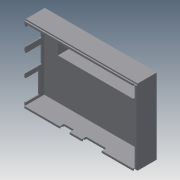
# Autodesk Inventor part: raspi_enclosure2
Saved by Autodesk Inventor 2015 (Build 190159000, 159)
## iProperties
Created: 2018-01-16
Part Number: raspi_enclosure2
Material: Generic
Document SubType Name: Modeling
Designer: rissa
Density: 1 g/cm^3
Appearance: Default
Author: rissa
Autodesk Inventor part; units mm, degrees
ref_plane "YZ Plane" through (0, 0, 0) normal (1, 0, 0) x (0, 1, 0)
ref_plane "XZ Plane" through (0, 0, 0) normal (0, 1, 0) x (-1, 0, 0)
ref_plane "XY Plane" through (0, 0, 0) normal (0, 0, 1) x (1, 0, 0)
sketch "Sketch1" plane through (0, 0, 0) normal (0, 0, 1) x (1, 0, 0)
  line L0 (-43.7903, 41.0199) -> (46.7097, 41.0199)
  line L1 (46.7097, 41.0199) -> (46.7097, -19.9801)
  line L2 (46.7097, -19.9801) -> (-43.7903, -19.9801)
  line L3 (-43.7903, -19.9801) -> (-43.7903, 41.0199)
  point P0 (0, 0)
  dimension "d0" = 90.5
  dimension "d1" = 61
  constraints: 8 end point, 2 parallel, 1 horizontal, 1 perpendicular
  measures "d0" distance of L0.start L0.end
  measures "d1" distance between parallel lines of L2 L0
extrude "Extrusion1" add sketch "Sketch1" along normal blind 1.5
sketch "Sketch2" plane through (0, 0, 1.5) normal (0, 0, 1) x (1, 0, 0)
  line L0 (-42.7903, 39.5199) -> (45.2097, 39.5199)
  line L1 (45.2097, 39.5199) -> (45.2097, -18.4801)
  line L2 (45.2097, -18.4801) -> (-42.7903, -18.4801)
  line L3 (-42.7903, -18.4801) -> (-42.7903, 39.5199)
  line L4 (-43.7903, 41.0199) -> (46.7097, 41.0199)
  line L5 (46.7097, 41.0199) -> (46.7097, -19.9801)
  line L6 (46.7097, -19.9801) -> (-43.7903, -19.9801)
  line L7 (-43.7903, -19.9801) -> (-43.7903, 41.0199)
  point P0 (0, 0)
  dimension "d4" = 1.5
  dimension "d5" = 1.5
  dimension "d6" = 1.5
  dimension "d7" = 1
  constraints: 16 end point, 4 parallel, 2 horizontal, 2 perpendicular
  measures "d4" distance between parallel lines of L4 L0
  measures "d5" distance between parallel lines of L5 L1
  measures "d6" distance between parallel lines of L6 L2
  measures "d7" distance between parallel lines of L3 L7
extrude "Extrusion2" add sketch "Sketch2" along normal blind 16
sketch "Sketch3" plane through (-43.7903, -19.9801, 0) normal (-1, 0, 0) x (0, 0, 1)
  line L0 (17.5, 1.5) -> (17.5, 59.5) projected
  line L1 (17.5, 20.5) -> (5.5, 20.5)
  line L2 (5.5, 20.5) -> (5.5, 3.5)
  line L3 (5.5, 3.5) -> (17.5, 3.5)
  line L4 (17.5, 3.5) -> (17.5, 20.5)
  line L5 (17.5, 38) -> (3.5, 38)
  line L6 (3.5, 38) -> (3.5, 24)
  line L7 (3.5, 24) -> (17.5, 24)
  line L8 (17.5, 24) -> (17.5, 38)
  line L9 (17.5, 56.5) -> (3.5, 56.5)
  line L10 (3.5, 56.5) -> (3.5, 42.5)
  line L11 (3.5, 42.5) -> (17.5, 42.5)
  line L12 (17.5, 42.5) -> (17.5, 56.5)
  line L13 (0, 0) -> (17.5, 0) projected
  point P0 (0, 19.9801)
  dimension "d10" = 3.5
  dimension "d11" = 12
  dimension "d12" = 17
  dimension "d13" = 3.5
  dimension "d14" = 14
  dimension "d15" = 14
  dimension "d16" = 14
  dimension "d17" = 4.5
  dimension "d18" = 14
  constraints: 24 end point, 6 parallel, 3 horizontal, 3 perpendicular, 3 point on line
  measures "d10" distance between parallel lines of L13 L3
  measures "d11" distance between parallel lines of L2 L0
  measures "d12" distance between parallel lines of L3 L1
  measures "d13" distance between parallel lines of L7 L1
  measures "d14" distance between parallel lines of L8 L6
  measures "d15" distance between parallel lines of L7 L5
  measures "d16" distance between parallel lines of L11 L9
  measures "d17" distance between parallel lines of L5 L11
  measures "d18" distance between parallel lines of L0 L10
extrude "Extrusion3" cut sketch "Sketch3" against normal blind 1
sketch "Sketch4" plane through (0, 0, 1.5) normal (0, 0, 1) x (1, 0, 0)
  line L0 (45.2097, 39.5199) -> (-15.7903, 39.5199)
  line L1 (-15.7903, 39.5199) -> (-15.7903, 30.5199)
  line L2 (-15.7903, 30.5199) -> (45.2097, 30.5199)
  line L3 (45.2097, 30.5199) -> (45.2097, 39.5199)
  point P0 (0, 0)
  dimension "d21" = 61
  dimension "d22" = 9
  constraints: 8 end point, 2 parallel, 1 horizontal, 1 perpendicular
  measures "d21" distance between parallel lines of L1 L3
  measures "d22" distance between parallel lines of L0 L2
extrude "Extrusion4" cut sketch "Sketch4" against normal blind 1.5
sketch "Sketch5" plane through (0, 0, 1.5) normal (0, 0, 1) x (1, 0, 0)
  line L0 (45.2097, 30.5199) -> (-15.7903, 30.5199)
  line L1 (-15.7903, 30.5199) -> (-15.7903, 29.0199)
  line L2 (-15.7903, 29.0199) -> (45.2097, 29.0199)
  line L3 (45.2097, 29.0199) -> (45.2097, 30.5199)
  line L4 (-42.7903, 39.5199) -> (45.2097, 39.5199) projected
  line L5 (-15.7903, 29.0199) -> (-17.2903, 29.0199)
  line L6 (-17.2903, 29.0199) -> (-17.2903, 39.5199)
  line L7 (-17.2903, 39.5199) -> (-15.7903, 39.5199)
  line L8 (-15.7903, 39.5199) -> (-15.7903, 29.0199)
  line L9 (46.7097, 41.0199) -> (46.7097, -19.9801) projected
  line L10 (45.2097, -18.4801) -> (45.2097, 30.5199) projected
  point P0 (0, 0)
  dimension "d25" = 1.5
  dimension "d26" = 1.5
  dimension "d28" = 61
  dimension "d29" = 9
  constraints: 16 end point, 4 parallel, 2 horizontal, 2 perpendicular, 1 point on line
  measures "d25" distance between parallel lines of L2 L0
  measures "d26" distance between parallel lines of L8 L6
  measures "d28" distance between parallel lines of L8 L10
  measures "d29" distance between parallel lines of L4 L0
extrude "Extrusion5" add sketch "Sketch5" along normal blind 16
sketch "Sketch6" plane through (0, 0, 17.5) normal (0, 0, 1) x (1, 0, 0)
  line L0 (-43.7903, 0.5199) -> (-42.7903, 0.5199) projected
  line L1 (-42.7903, 4.0199) -> (-43.7903, 4.0199) projected
  line L2 (-42.7903, 0.5199) -> (-42.7903, 4.0199) projected
  line L3 (-43.7903, 4.0199) -> (-43.7903, 0.5199) projected
  line L4 (-43.7903, -19.9801) -> (-43.7903, 41.0199) projected
  line L5 (-43.2903, 4.0199) -> (-43.7903, 4.0199)
  line L6 (-43.7903, 4.0199) -> (-43.7903, 3.0199)
  line L7 (-43.7903, 3.0199) -> (-43.2903, 3.0199)
  line L8 (-43.2903, 3.0199) -> (-43.2903, 4.0199)
  point P0 (0, 0)
  dimension "d32" = 3.5
  dimension "d33" = 1
  dimension "d34" = 0.5
  dimension "d35" = 1
  constraints: 8 end point, 2 parallel, 1 horizontal, 1 midpoint, 1 perpendicular, 1 point on line
  measures "d32" distance between parallel lines of L0 L1
  measures "d33" distance between parallel lines of L2 L3
  measures "d34" distance between parallel lines of L8 L3
  measures "d35" distance between parallel lines of L1 L7
extrude "Extrusion6" cut sketch "Sketch6" against normal blind 12 contours L3 L1 L8 L7
sketch "Sketch7" plane through (0, 0, 17.5) normal (0, 0, 1) x (1, 0, 0)
  line L0 (-43.7903, 18.0199) -> (-42.7903, 18.0199) projected
  line L1 (-43.7903, 22.5199) -> (-43.7903, 18.0199) projected
  line L2 (-43.2903, 18.0199) -> (-43.7903, 18.0199)
  line L3 (-43.7903, 18.0199) -> (-43.7903, 19.0199)
  line L4 (-43.7903, 19.0199) -> (-43.2903, 19.0199)
  line L5 (-43.2903, 19.0199) -> (-43.2903, 18.0199)
  point P0 (0, 0)
  dimension "d38" = 1
  constraints: 8 end point, 2 parallel, 1 horizontal, 1 midpoint, 1 perpendicular, 1 point on line
  measures "d38" distance from line of L3.end L0
extrude "Extrusion7" cut sketch "Sketch7" against normal blind 12
sketch "Sketch8" plane through (0, 0, 17.5) normal (0, 0, 1) x (1, 0, 0)
  line L0 (-43.7903, 22.5199) -> (-43.7903, 19.0199) projected
  line L1 (-43.2903, 22.5199) -> (-43.7903, 22.5199)
  line L2 (-43.7903, 22.5199) -> (-43.7903, 21.5199)
  line L3 (-43.7903, 21.5199) -> (-43.2903, 21.5199)
  line L4 (-43.2903, 21.5199) -> (-43.2903, 22.5199)
  line L5 (-42.7903, 22.5199) -> (-43.7903, 22.5199) projected
  point P0 (0, 0)
  dimension "d41" = 0.5
  dimension "d42" = 1
  dimension "d43" = 1
  constraints: 8 end point, 2 parallel, 1 horizontal, 1 perpendicular, 1 point on line
  measures "d41" distance between parallel lines of L4 L0
  measures "d42" distance from line of L3 L1.start
  measures "d43" distance between parallel lines of L3 L5
extrude "Extrusion8" cut sketch "Sketch8" against normal blind 12
sketch "Sketch9" plane through (0, 0, 17.5) normal (0, 0, 1) x (1, 0, 0)
  line L0 (-43.7903, 36.5199) -> (-42.7903, 36.5199) projected
  line L1 (-43.7903, 41.0199) -> (-43.7903, 36.5199) projected
  line L2 (-43.2903, 36.5199) -> (-43.7903, 36.5199)
  line L3 (-43.7903, 36.5199) -> (-43.7903, 37.5199)
  line L4 (-43.7903, 37.5199) -> (-43.2903, 37.5199)
  line L5 (-43.2903, 37.5199) -> (-43.2903, 36.5199)
  point P0 (0, 0)
  dimension "d46" = 1
  dimension "d47" = 0.5
  constraints: 8 end point, 2 parallel, 1 horizontal, 1 midpoint, 1 perpendicular, 1 point on line
  measures "d46" distance between parallel lines of L0 L4
  measures "d47" distance between parallel lines of L1 L5
extrude "Extrusion9" cut sketch "Sketch9" against normal blind 12
sketch "Sketch10" plane through (-43.7903, -19.9801, 0) normal (0, -1, 0) x (1, 0, 0)
  line L0 (29.5, 17.5) -> (37.5, 17.5)
  line L1 (37.5, 17.5) -> (37.5, 14)
  line L2 (37.5, 14) -> (29.5, 14)
  line L3 (29.5, 14) -> (29.5, 17.5)
  line L4 (0, 0) -> (0, 17.5) projected
  line L5 (47.5, 17.5) -> (63.5, 17.5)
  line L6 (63.5, 17.5) -> (63.5, 14)
  line L7 (63.5, 14) -> (47.5, 14)
  line L8 (47.5, 14) -> (47.5, 17.5)
  line L9 (90.5, 0) -> (90.5, 17.5) projected
  point P0 (43.7903, 0)
  dimension "d50" = 29.5
  dimension "d51" = 8
  dimension "d53" = 16
  dimension "d57" = 10
  constraints: 16 end point, 4 parallel, 2 horizontal, 2 perpendicular
  measures "d50" distance between parallel lines of L3 L4
  measures "d51" distance between parallel lines of L1 L3
  measures "d53" distance between parallel lines of L6 L8
  measures "d57" distance between parallel lines of L8 L1
extrude "Extrusion10" cut sketch "Sketch10" against normal blind 1.5
sketch "Sketch11" plane through (-43.7903, -19.9801, 0) normal (0, -1, 0) x (1, 0, 0)
  line L0 (63.5, 17.5) -> (63.5, 14) projected
  line L1 (90.5, 0) -> (90.5, 17.5) projected
  line L2 (63.5, 16.6) -> (90.5, 16.6)
  line L3 (90.5, 16.6) -> (90.5, 15.5)
  line L4 (90.5, 15.5) -> (63.5, 15.5)
  line L5 (63.5, 15.5) -> (63.5, 16.6)
  line L6 (37.5, 17.5) -> (37.5, 14) projected
  line L7 (47.5, 14) -> (47.5, 17.5) projected
  line L8 (37.5, 16.6) -> (47.5, 16.6)
  line L9 (47.5, 16.6) -> (47.5, 15.5)
  line L10 (47.5, 15.5) -> (37.5, 15.5)
  line L11 (37.5, 15.5) -> (37.5, 16.6)
  line L12 (0, 0) -> (0, 17.5) projected
  line L13 (29.5, 14) -> (29.5, 17.5) projected
  line L14 (0, 16.6) -> (29.5, 16.6)
  line L15 (29.5, 16.6) -> (29.5, 15.5)
  line L16 (29.5, 15.5) -> (0, 15.5)
  line L17 (0, 15.5) -> (0, 16.6)
  line L18 (63.5, 17.5) -> (90.5, 17.5) projected
  line L19 (37.5, 17.5) -> (47.5, 17.5) projected
  line L20 (0, 17.5) -> (29.5, 17.5) projected
  point P0 (43.7903, 0)
  dimension "d61" = 1.1
  dimension "d62" = 0.9
  dimension "d63" = 1.1
  dimension "d64" = 0.9
  dimension "d65" = 1.1
  dimension "d66" = 0.9
  constraints: 24 end point, 6 parallel, 6 point on line, 3 horizontal, 3 perpendicular
  measures "d61" distance between parallel lines of L2 L4
  measures "d62" distance between parallel lines of L2 L18
  measures "d63" distance between parallel lines of L10 L8
  measures "d64" distance between parallel lines of L8 L19
  measures "d65" distance between parallel lines of L14 L16
  measures "d66" distance between parallel lines of L14 L20
extrude "Extrusion11" cut sketch "Sketch11" against normal blind 1 contours L2 L1 L4 L0 | L8 L7 L10 L6 | L12 L14 L13 L16
sketch "Sketch12" plane through (-43.7903, 41.0199, 0) normal (0, 1, 0) x (1, 0, 0)
  line L0 (90.5, 0) -> (90.5, -17.5) projected
  line L1 (0, 0) -> (0, -17.5) projected
  line L2 (90.5, -16.6) -> (0, -16.6)
  line L3 (0, -16.6) -> (0, -15.5)
  line L4 (0, -15.5) -> (90.5, -15.5)
  line L5 (90.5, -15.5) -> (90.5, -16.6)
  line L6 (90.5, -17.5) -> (0, -17.5) projected
  point P0 (43.7903, 0)
  dimension "d69" = 1.1
  dimension "d70" = 0.9
  constraints: 8 end point, 2 parallel, 2 point on line, 1 horizontal, 1 perpendicular
  measures "d69" distance between parallel lines of L4 L2
  measures "d70" distance between parallel lines of L6 L2
extrude "Extrusion12" cut sketch "Sketch12" against normal blind 1 contours L0 L2 L1 L4
sketch "Sketch13" plane through (0, 0, 17.5) normal (0, 0, 1) x (1, 0, 0)
  line L0 (-42.7903, -16.4801) -> (-43.7903, -16.4801)
  line L1 (-43.7903, -16.4801) -> (-43.7903, -19.9801)
  line L2 (-43.7903, -19.9801) -> (-42.7903, -19.9801)
  line L3 (-42.7903, -19.9801) -> (-42.7903, -16.4801)
  point P0 (0, 0)
  constraints: 8 end point, 2 parallel, 1 horizontal, 1 perpendicular
extrude "Extrusion13" cut sketch "Sketch13" against normal blind 1
sketch "Sketch14" plane through (0, 0, 17.5) normal (0, 0, 1) x (1, 0, 0)
  line L0 (-42.7903, 4.0199) -> (-43.7903, 4.0199)
  line L1 (-43.7903, 4.0199) -> (-43.7903, 0.5199)
  line L2 (-43.7903, 0.5199) -> (-42.7903, 0.5199)
  line L3 (-42.7903, 0.5199) -> (-42.7903, 4.0199)
  point P0 (0, 0)
  constraints: 8 end point, 2 parallel, 1 horizontal, 1 perpendicular
extrude "Extrusion14" cut sketch "Sketch14" against normal blind 1
sketch "Sketch15" plane through (0, 0, 17.5) normal (0, 0, 1) x (1, 0, 0)
  line L0 (-43.7903, 21.5199) -> (-43.7903, 19.0199) projected
  line L1 (-42.7903, 22.5199) -> (-43.7903, 22.5199)
  line L2 (-43.7903, 22.5199) -> (-43.7903, 20.2699)
  line L3 (-43.7903, 20.2699) -> (-42.7903, 20.2699)
  line L4 (-42.7903, 20.2699) -> (-42.7903, 22.5199)
  line L5 (-42.7903, 18.0199) -> (-43.7903, 18.0199)
  line L6 (-43.7903, 18.0199) -> (-43.7903, 20.2699)
  line L7 (-43.7903, 20.2699) -> (-42.7903, 20.2699)
  line L8 (-42.7903, 20.2699) -> (-42.7903, 18.0199)
  point P0 (0, 0)
  constraints: 16 end point, 4 parallel, 2 horizontal, 2 perpendicular, 1 midpoint
extrude "Extrusion15" cut sketch "Sketch15" against normal blind 1
sketch "Sketch16" plane through (0, 0, 17.5) normal (0, 0, 1) x (1, 0, 0)
  line L0 (-43.7903, 41.0199) -> (-42.7903, 41.0199)
  line L1 (-42.7903, 41.0199) -> (-42.7903, 36.5199)
  line L2 (-42.7903, 36.5199) -> (-43.7903, 36.5199)
  line L3 (-43.7903, 36.5199) -> (-43.7903, 41.0199)
  point P0 (0, 0)
  constraints: 8 end point, 2 parallel, 1 horizontal, 1 perpendicular
extrude "Extrusion16" cut sketch "Sketch16" against normal blind 1
sketch "Sketch17" plane through (0, 0, 17.5) normal (0, 0, 1) x (1, 0, 0)
  line L0 (46.7097, -19.9801) -> (45.0097, -19.9801)
  line L1 (45.0097, -19.9801) -> (45.0097, 41.0199)
  line L2 (45.0097, 41.0199) -> (46.7097, 41.0199)
  line L3 (46.7097, 41.0199) -> (46.7097, -19.9801)
  point P0 (0, 0)
  dimension "d81" = 61
  dimension "d84" = 1.7
  constraints: 8 end point, 2 parallel, 1 horizontal, 1 perpendicular
  measures "d81" distance from line of L0.start L2
  measures "d84" distance between parallel lines of L1 L3
extrude "Extrusion17" cut sketch "Sketch17" against normal blind 1
body "Solid1"
